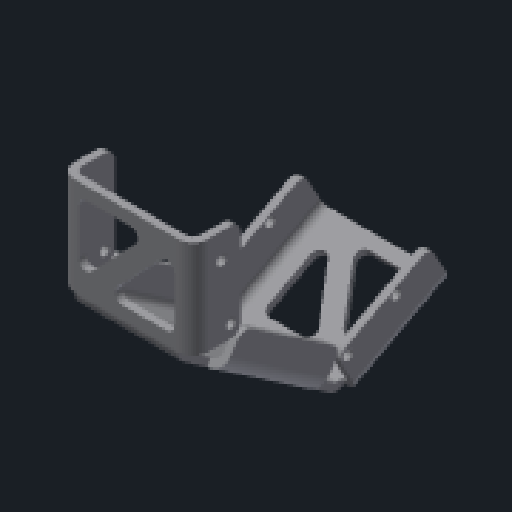
# Autodesk Inventor part: HipCoverTop
Saved by Autodesk Inventor 2025.2 (Build 292293000, 293)
## iProperties
Created: 2020-05-24
Part Number: HipCoverTop
Material: Generic
Document SubType Name: Sheet Metal
Designer: valer
Density: 1 g/cm^3
Sheet Metal Rule: Default
Appearance: Default
Author: valer
Autodesk Inventor part; units mm, degrees
ref_plane "YZ Plane" through (0, 0, 0) normal (1, 0, 0) x (0, 1, 0)
ref_plane "XZ Plane" through (0, 0, 0) normal (0, 1, 0) x (-1, 0, 0)
ref_plane "XY Plane" through (0, 0, 0) normal (0, 0, 1) x (1, 0, 0)
sketch "Base" plane through (0, 0, 0) normal (0, 0, 1) x (1, 0, 0)
  line L0 (0, 0) -> (44.5, 0)
  line L1 (44.5, 0) -> (44.5, -65.2018)
  line L2 (44.5, -65.2018) -> (0, -65.2018)
  line L3 (0, -65.2018) -> (0, 0)
  dimension "d0" = 65.2018
  dimension "d1" = 44.5
  measures "d0" distance of L2.end L0.start
  measures "d1" distance of L0.start L0.end
extrude "Plate1" add sketch "Base" along normal blind 5
sketch "Sketch2" plane through (5, 0, 5) normal (-1, 0, 0) x (0, -1, 0)
  line L0 (65.2018, 0) -> (0, 0)
  line L1 (0, 0) -> (0, -31.75)
  line L2 (0, -31.75) -> (65.2018, -31.75)
  line L3 (65.2018, -31.75) -> (65.2018, 0)
  constraints: 6 end point, 1 horizontal, 1 perpendicular, 1 vertical
edge flange "MountFeature" height 31.75 angle 90 thickness 5 bend radius 5 thickness toward (-1, 0, 0) relief straight relief width 5 relief depth 2.5 edges at (0, -32.6009, 0) wall of the first edge with corners at (5, -65.2018, 5) (5, 0, 5) (5, 0, -26.75) (5, -65.2018, -26.75)
bend "Bend1"
corner "Corner1"
sketch "MountHoles" plane through (0, -65.2018, -26.75) normal (-1, 0, 0) x (0, 0, 1)
  arc A0 (10.1508, 50.0369) -> (15.4938, 46.6054) centre (12.8223, 48.3211) ccw projected
  arc A1 (7.8027, 11.5289) -> (5.1061, 5.7799) centre (6.4544, 8.6544) ccw projected
hole "MountHolesFeature" at (0, -16.8807, -13.9277) at (0, -56.5474, -20.2956) direction (1, 0, 0) diameter 6.35 end through all
mirror "MirrorFeature" about plane through (44.5, 0, 0) normal (1, 0, 0)
sketch "GenerativeCut1" plane through (0, 0, 5) normal (0, 0, 1) x (1, 0, 0)
  line L0 (12.7, -8.4667) -> (12.7, -56.7351)
  line L1 (12.7, -56.7351) -> (58.7478, -8.4667)
  line L2 (58.7478, -8.4667) -> (12.7, -8.4667)
  line L3 (79, 0) -> (10, 0) projected
  line L4 (30.2522, -56.7351) -> (76.3, -8.4667)
  line L5 (76.3, -8.4667) -> (76.3, -56.7351)
  line L6 (76.3, -56.7351) -> (30.2522, -56.7351)
  line L7 (58.7478, -8.4667) -> (76.3, -8.4667) construction
  line L8 (12.7, -56.7351) -> (30.2522, -56.7351) construction
  line L9 (0, -65.2018) -> (0, 0) projected
  line L10 (89, -65.2018) -> (89, 0) projected
  line L11 (79, -65.2018) -> (10, -65.2018) projected
  dimension "d23" = 8.4667
  dimension "d24" = 12.7
  dimension "d25" = 12.7
  dimension "d26" = 8.4667
  dimension "d27" = 12.7
  constraints: 16 end point, 2 parallel, 2 perpendicular, 1 collinear, 1 horizontal, 1 vertical
  measures "d23" distance between parallel lines of L3 L2
  measures "d24" distance between parallel lines of L9 L0
  measures "d25" distance between parallel lines of L5 L10
  measures "d26" distance between parallel lines of L11 L6
  measures "d27" distance between parallel lines of L4 L1
extrude "GenerativeCut1Feature" cut sketch "GenerativeCut1" against normal blind 25.4
fillet "GenerativeCut1FilletsFeature" radius 5.08 6 edges at (12.7, -8.4667, 2.5) (12.7, -56.7351, 2.5) (58.7478, -8.4667, 2.5) (76.3, -8.4667, 2.5) (30.2522, -56.7351, 2.5) (76.3, -56.7351, 2.5)
sketch "Sketch5" plane through (79, -69.3397, -2.1932) normal (0, -0.8275708, 0.5613614) x (1, 0, 0)
  line L0 (-69, 0) -> (0, 0)
  line L1 (0, 0) -> (0, 116.6197)
  line L2 (0, 116.6197) -> (-69, 116.6197)
  line L3 (-69, 116.6197) -> (-69, 0)
  constraints: 6 end point, 1 horizontal, 1 perpendicular, 1 vertical
edge flange "KneeFlangeFeature" height 121.92 angle 55.85 thickness 5 bend radius 5 thickness toward (0, -0.8275708, 0.5613614) relief straight relief width 5 relief depth 2.5 edges at (44.5, -65.2018, 5) wall of the first edge with corners at (10, -69.3397, -2.1932) (79, -69.3397, -2.1932) (79, -134.8054, -98.7042) (10, -134.8054, -98.7042)
bend "Bend2"
corner "Corner2"
sketch "Sketch6" plane through (10, -135.0807, -103.8615) normal (0, -0.8826196, -0.4700879) x (1, 0, 0)
  line L0 (69, 0) -> (0, 0)
  line L1 (0, 0) -> (0, -70.1688)
  line L2 (0, -70.1688) -> (69, -70.1688)
  line L3 (69, -70.1688) -> (69, 0)
  constraints: 6 end point, 1 horizontal, 1 perpendicular, 1 vertical
edge flange "KneeBottomFlangeFeature" height 76.2 angle 62.19 thickness 5 bend radius 5 thickness toward (0, -0.8826196, -0.4700879) relief straight relief width 5 relief depth 2.5 edges at (44.5, -134.8054, -98.7042) wall of the first edge with corners at (79, -135.0807, -103.8615) (10, -135.0807, -103.8615) (10, -102.0952, -165.7938) (79, -102.0952, -165.7938)
bend "Bend3"
corner "Corner3"
sketch "Sketch8" plane through (5, -130.6676, -101.511) normal (-1, 0, 0) x (0, -1, 0)
  line L0 (-32.9855, -61.9324) -> (0, 0)
  line L1 (0, 0) -> (-19.197, 10.2244)
  line L2 (-19.197, 10.2244) -> (-52.1825, -51.708)
  line L3 (-52.1825, -51.708) -> (-32.9855, -61.9324)
  constraints: 6 end point, 1 perpendicular, 2 other
edge flange "KneeBottomSidesFeature" height 31.75 angle 90 thickness 5 bend radius 5 thickness toward (-1, 0, 0) relief straight relief width 5 relief depth 2.5 corner gap 5 corner form 0 edges at (10, -118.5879, -134.8277) (79, -118.5879, -134.8277) wall of the first edge with corners at (5, -97.6821, -163.4434) (5, -130.6676, -101.511) (5, -111.4706, -91.2866) (5, -78.4851, -153.219)
bend "Bend4"
corner "Corner4"
fillet "OutsideFilletsFeature" radius 6.35 8 edges at (2.5, -65.2018, -26.75) (2.5, 0, -26.75) (2.5, -111.4706, -91.2866) (86.5, -78.4851, -153.219) (2.5, -78.4851, -153.219) (86.5, -111.4706, -91.2866) (86.5, -65.2018, -26.75) (86.5, 0, -26.75)
sketch "Sketch10" plane through (10, -73.4775, 0.6136) normal (0, -0.8275708, 0.5613614) x (1, 0, 0)
  line L0 (-5, -15.5299) -> (-10, -15.5299) projected
  line L1 (-5, -99.6109) -> (-10, -99.6109) projected
  line L2 (-10, -18.0699) -> (0, -18.0699)
  line L3 (0, -18.0699) -> (0, -97.0709)
  line L4 (0, -97.0709) -> (-10, -97.0709)
  line L5 (-10, -97.0709) -> (-10, -18.0699)
  line L6 (-10, 0) -> (-10, -12.7446) projected
  line L7 (0, 0) -> (0, -116.6197) projected
  point P0 (-10, 40.7396)
  dimension "d65" = 2.54
  dimension "d66" = 2.54
  constraints: 8 end point, 2 collinear, 2 parallel, 1 horizontal, 1 perpendicular
  measures "d65" distance between parallel lines of L0 L2
  measures "d66" distance between parallel lines of L1 L4
sheet face with bend "SideFlangeBaseFeature" sketch "Sketch10" thickness 5 toward (0, 0.8275708, -0.5613614) bend radius 5 relief straight relief width 5 relief depth 2.5
bend "Bend5"
sketch "Sketch11" plane through (5, -83.6213, -14.3405) normal (-1, 0, 0) x (0, -1, 0)
  line L0 (44.3481, -65.3789) -> (0, 0)
  line L1 (0, 0) -> (-21.0203, -14.2586)
  line L2 (-21.0203, -14.2586) -> (23.3278, -79.6375)
  line L3 (23.3278, -79.6375) -> (44.3481, -65.3789)
  constraints: 6 end point, 1 perpendicular, 2 other
edge flange "SideFlangeFeature" height 25.4 angle 90 thickness 5 bend radius 5 thickness toward (-1, 0, 0) relief straight relief width 5 relief depth 2.5 edges at (0, -101.6575, -49.8368) wall of the first edge with corners at (5, -127.9694, -79.7194) (5, -83.6213, -14.3405) (5, -62.601, -28.5991) (5, -106.9491, -93.978)
bend "Bend6"
corner "Corner5"
ref_plane "MiddlePlane" through (44.5, -97.6821, -163.4434) normal (-1, 0, 0) x (0, -0.4700879, 0.8826196)
mirror "SideFlangeMirrorFeature" about plane through (44.5, -97.6821, -163.4434) normal (-1, 0, 0) of "SideFlangeFeature"
fillet "SideFlangeFilletsFeature" radius 6.35 4 edges at (2.5, -106.9491, -93.978) (86.5, -106.9491, -93.978) (2.5, -62.601, -28.5991) (86.5, -62.601, -28.5991)
sketch "KneeMountHoles" plane through (0, -97.6821, -163.4434) normal (-1, 0, 0) x (0, -0.4700879, 0.8826196)
  arc A0 (30.8237, 17.3045) -> (24.5578, 18.3345) centre (27.6908, 17.8195) ccw projected
  arc A1 (68.2036, 17.5356) -> (62.1887, 15.4999) centre (65.1961, 16.5177) ccw projected
  point P0 (98.3392, 163.0489)
hole "KneeMountHolesFeature" at (0, -113.7511, -98.1352) at (0, -94.9714, -130.6263) direction (1, 0, 0) diameter 6.35 end through all
sketch "Rais" plane through (10, -73.4775, 0.6136) normal (0, -0.8275708, 0.5613614) x (1, 0, 0)
  line L0 (69, 0) -> (0, 0) construction
  line L1 (0, -116.6197) -> (69, -116.6197) construction
  line L2 (0, 0) -> (69, 0) construction
  line L3 (34.5, 0) -> (34.5, -116.6197) construction
  line L4 (0, -116.6197) -> (69, -116.6197) construction
  line L5 (26.2901, -42.5901) -> (17.3099, -33.6099) construction
  line L6 (24.0451, -44.8352) -> (15.0648, -35.8549)
  line L7 (19.5549, -31.3648) -> (28.5352, -40.3451)
  arc A0 (24.0451, -44.8352) -> (28.5352, -40.3451) centre (26.2901, -42.5901) ccw
  arc A1 (19.5549, -31.3648) -> (15.0648, -35.8549) centre (17.3099, -33.6099) ccw
  line L8 (0, -18.0699) -> (0, -97.0709) construction
  line L9 (0, -57.5704) -> (69, -57.5704) construction
  line L10 (69, -97.0709) -> (69, -18.0699) construction
  line L11 (44.9549, -44.8352) -> (53.9352, -35.8549)
  line L12 (49.4451, -31.3648) -> (40.4648, -40.3451)
  arc A2 (40.4648, -40.3451) -> (44.9549, -44.8352) centre (42.7099, -42.5901) ccw
  arc A3 (53.9352, -35.8549) -> (49.4451, -31.3648) centre (51.6901, -33.6099) ccw
  line L13 (24.0451, -70.3057) -> (15.0648, -79.2859)
  line L14 (19.5549, -83.7761) -> (28.5352, -74.7958)
  arc A4 (28.5352, -74.7958) -> (24.0451, -70.3057) centre (26.2901, -72.5507) ccw
  arc A5 (15.0648, -79.2859) -> (19.5549, -83.7761) centre (17.3099, -81.531) ccw
  line L15 (44.9549, -70.3057) -> (53.9352, -79.2859)
  arc A6 (49.4451, -83.7761) -> (53.9352, -79.2859) centre (51.6901, -81.531) ccw
  line L16 (49.4451, -83.7761) -> (40.4648, -74.7958)
  arc A7 (44.9549, -70.3057) -> (40.4648, -74.7958) centre (42.7099, -72.5507) ccw
  point P0 (-10, 40.7396)
  point P1 (21.8, -38.1)
  dimension "d101" = 3.175
  dimension "d102" = 12.7
  dimension "d103" = 12.7
  dimension "d104" = 38.1
  dimension "d105" = 45
  constraints: 24 end point, 18 symmetric about line, 16 point on circle, 8 centre point, 5 midpoint, 4 tangent, 1 parallel, 6 other
  measures "d101" radius of A1
  measures "d102" distance from line of L3 point (21.8, -38.1)
  measures "d103" distance of L5.start L5.end
  measures "d104" distance from line of L0 point (21.8, -38.1)
  measures "d105" angle of L3 L5
extrude "RailsFeature" cut sketch "Rais" against normal blind 25.4
sketch "GenerativeCut2" plane through (10, -139.4938, -106.2119) normal (0, -0.8826196, -0.4700879) x (1, 0, 0)
  line L0 (8.4667, -8.4667) -> (8.4667, -61.7021)
  line L1 (8.4667, -61.7021) -> (45.1149, -8.4667)
  line L2 (45.1149, -8.4667) -> (8.4667, -8.4667)
  line L3 (23.8851, -61.7021) -> (60.5333, -8.4667)
  line L4 (60.5333, -8.4667) -> (60.5333, -61.7021)
  line L5 (60.5333, -61.7021) -> (23.8851, -61.7021)
  line L6 (45.1149, -8.4667) -> (60.5333, -8.4667) construction
  line L7 (8.4667, -61.7021) -> (23.8851, -61.7021) construction
  line L8 (69, 0) -> (0, 0) projected
  line L9 (0, -70.1688) -> (0, 0) projected
  line L10 (69, -70.1688) -> (0, -70.1688) projected
  line L11 (69, 0) -> (69, -70.1688) projected
  point P0 (-10, 28.1704)
  dimension "d124" = 12.7
  dimension "d125" = 8.4667
  dimension "d126" = 8.4667
  dimension "d127" = 8.4667
  dimension "d128" = 8.4667
  constraints: 16 end point, 2 perpendicular, 1 collinear, 1 horizontal, 1 parallel, 1 vertical
  measures "d124" distance between parallel lines of L3 L1
  measures "d125" distance between parallel lines of L8 L2
  measures "d126" distance between parallel lines of L9 L0
  measures "d127" distance between parallel lines of L11 L4
  measures "d128" distance between parallel lines of L10 L5
extrude "GenerativeCut2Feature" cut sketch "GenerativeCut2" against normal blind 25.4 contours L2 L1 L0 | L3 L4 L5
fillet "GenerativeCut2FilletsFeature" radius 5.08 6 edges at (18.4667, -133.3072, -112.5095) (55.1149, -133.3072, -112.5095) (18.4667, -108.2818, -159.4962) (33.8851, -108.2818, -159.4962) (70.5333, -133.3072, -112.5095) (70.5333, -108.2818, -159.4962)
equation "\"d20\" = Thickness"
equation "\"d25\" = d24"
equation "\"d26\" = d23"
equation "\"d27\" = d24"
equation "\"d88\" = Thickness"
equation "\"d124\" = d121"
equation "\"d2\" = Thickness"
equation "\"d3\" = BendReliefWidth"
equation "\"d4\" = BendReliefDepth"
equation "\"d5\" = MinimumRemnant"
equation "\"d6\" = TransitionRadius"
equation "\"d9\" = BendRadius"
equation "\"d10\" = CornerReliefSize"
equation "\"d11\" = GapSize"
equation "\"d12\" = JacobiRadiusSize"
equation "\"d31\" = BendReliefWidth"
equation "\"d32\" = BendReliefDepth"
equation "\"d33\" = MinimumRemnant"
equation "\"d34\" = TransitionRadius"
equation "\"d37\" = BendRadius"
equation "\"d38\" = CornerReliefSize"
equation "\"d39\" = GapSize"
equation "\"d40\" = JacobiRadiusSize"
equation "\"d41\" = BendReliefWidth"
equation "\"d42\" = BendReliefDepth"
equation "\"d43\" = MinimumRemnant"
equation "\"d44\" = TransitionRadius"
equation "\"d47\" = BendRadius"
equation "\"d48\" = CornerReliefSize"
equation "\"d49\" = GapSize"
equation "\"d50\" = JacobiRadiusSize"
equation "\"d51\" = BendReliefWidth"
equation "\"d52\" = BendReliefDepth"
equation "\"d53\" = MinimumRemnant"
equation "\"d54\" = TransitionRadius"
equation "\"d57\" = BendRadius"
equation "\"d58\" = CornerReliefSize"
equation "\"d59\" = GapSize"
equation "\"d60\" = JacobiRadiusSize"
equation "\"d66\" = d65"
equation "\"d67\" = BendRadius"
equation "\"d68\" = BendReliefWidth"
equation "\"d70\" = MinimumRemnant"
equation "\"d69\" = BendReliefDepth"
equation "\"d71\" = TransitionRadius"
equation "\"d72\" = BendReliefWidth"
equation "\"d73\" = BendReliefDepth"
equation "\"d74\" = MinimumRemnant"
equation "\"d75\" = TransitionRadius"
equation "\"d78\" = BendRadius"
equation "\"d79\" = CornerReliefSize"
equation "\"d80\" = GapSize"
equation "\"d81\" = JacobiRadiusSize"
equation "\"BendRadius\" = Thickness"
equation "\"BendReliefWidth\" = Thickness"
equation "\"BendReliefDepth\" = 0.5 * Thickness"
equation "\"TransitionRadius\" = BendRadius"
equation "\"JacobiRadiusSize\" = BendRadius"
equation "\"GapSize\" = Thickness"
equation "\"Thickness\" = 5"
equation "\"d121\" = 12.7"
equation "\"MinimumRemnant\" = 10"
equation "\"CornerReliefSize\" = 20"
body "Solid1"
